Display Board 2 Mount (Autodesk Fusion 360 design; units mm, degrees)
Autodesk Fusion 360 part; units mm, degrees
sketch "Sketch1" plane through (0, 0, 0) normal (0, 0, 1) x (1, 0, 0)
  line L0 (-65.2, 0) -> (-65.2, 56.7)
  line L1 (0, 56.7) -> (0, 0)
  line L2 (3, -3) -> (-68.2, -3)
  line L3 (-68.2, -3) -> (-68.2, 59.7)
  line L4 (-68.2, 59.7) -> (3, 59.7)
  line L5 (3, 59.7) -> (3, -3)
  line L6 (-62.2, 59.7) -> (-62.2, 56.7)
  line L7 (-62.2, 0) -> (-62.2, -3)
  line L8 (-3, -3) -> (-3, 0)
  line L9 (-3, 56.7) -> (-3, 59.7)
  line L10 (-65.2, 56.7) -> (-62.2, 56.7)
  line L11 (-3, 56.7) -> (0, 56.7)
  line L12 (0, 0) -> (-3, 0)
  line L13 (-62.2, 0) -> (-65.2, 0)
  dimension "d1" = 65.2
  dimension "d2" = 56.7
  dimension "d4" = 6
  dimension "d5" = 6
  dimension "d6" = 6
  dimension "d7" = 6
  constraint horizontal L12
  constraint vertical L0
  constraint horizontal L10
  constraint vertical L1
  constraint coincident L1.end L12.start
  constraint coincident L4 L6.start
  constraint perpendicular L6 L10
  constraint coincident L7.start L12
  constraint coincident L2 L7.end
  constraint perpendicular L2 L7
  constraint coincident L2 L8.start
  constraint perpendicular L8 L12
  constraint coincident L9.start L10
  constraint coincident L4 L9.end
  constraint perpendicular L4 L9
  constraint collinear L10 L11
  constraint parallel L2 L12
  constraint parallel L0 L3
  constraint parallel L1 L5
  constraint collinear L12 L13
  measures "d1" distance of L1.end L0.start
  measures "d2" distance of L1.end L1.start
  measures "d4" distance of L5 L9
  measures "d5" distance of L3 L6
  measures "d6" distance of L3 L7
  measures "d7" distance of L5 L8
extrude "Extrude1" add sketch "Sketch1" along normal blind 6 contours L0 L2 L3 L4 L6 L7 L10 L13 | L1 L2 L4 L5 L8 L9 L11 L12 makes body 1 at (-68.2, 17.9, 2) makes body 2 at (3, 38.8, 2)
extrude "Extrude2" add sketch "Sketch1" along normal blind 3 contours L0 L1 L2 L4 L6 L7 L8 L9 L10 L11 L12 L13 bodies 1 2
